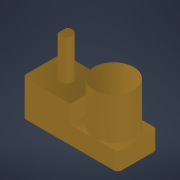
# Autodesk Inventor part: GM1024BY10
Saved by Autodesk Inventor 2022 (Build 260153000, 153)
## iProperties
Created: 2022-04-03
Part Number: GM1024BY10
Material: Bronze, Soft Tin
Document SubType Name: Modeling
Designer: Vinicius Miguel
Density: 8.874 g/cm^3
Appearance: Brass - Satin
Author: Vinicius Miguel
Autodesk Inventor part; units mm, degrees
ref_plane "YZ Plane" through (0, 0, 0) normal (1, 0, 0) x (0, 1, 0)
ref_plane "XZ Plane" through (0, 0, 0) normal (0, 1, 0) x (-1, 0, 0)
ref_plane "XY Plane" through (0, 0, 0) normal (0, 0, 1) x (1, 0, 0)
sketch "Sketch1" plane through (0, 0, 0) normal (0, 1, 0) x (-1, 0, 0)
  circle A0 centre (0, 0) radius 1.5
  dimension "d0" = 3
  constraints: 1 centre point, 1 coincident
  measures "d0" diameter of A0
extrude "Extrusion1" add sketch "Sketch1" along normal blind 10
sketch "Sketch2" plane through (0, 0, 0) normal (0, -1, 0) x (1, 0, 0)
  line L0 (6, 5) -> (-6, 5)
  line L1 (-6, 5) -> (-6, -5)
  line L2 (-6, -5) -> (6, -5)
  line L3 (6, -5) -> (6, 5)
  line L4 (6, 5) -> (-6, -5) construction
  line L5 (-6, 5) -> (6, -5) construction
  point P0 (0, 0)
  point P1 (0, 0)
  point P2 (0, 0)
  point P3 (0, 0)
  dimension "d3" = 10
  dimension "d4" = 12
  constraints: 12 end point, 4 midpoint, 2 coincident, 2 parallel, 1 horizontal, 1 perpendicular
  measures "d3" distance of L0.end L1.end
  measures "d4" distance of L0.start L0.end
extrude "Extrusion2" add sketch "Sketch2" along normal blind 9
sketch "Sketch3" plane through (6, 0, 5) normal (1, 0, 0) x (0, 0, -1)
  line L0 (10, 0) -> (0, 0) projected
  line L1 (0, 0) -> (0, -9) projected
  line L2 (10, -9) -> (0, -9) projected
  line L3 (10, 0) -> (10, -9) projected
  line L4 (0, 0) -> (0, -9) projected
  line L5 (0, -4.5) -> (10, -4.5)
  line L6 (10, 0) -> (10, -9) projected
  point P0 (5, 0)
  point P1 (0, -4.5)
  constraints: 2 end point, 2 midpoint
extrude "Extrusion3" add sketch "Sketch3" along normal blind 12 contours L3 L2 L1 L5
sketch "Sketch4" plane through (6, -4.5, 5) normal (0, 1, 0) x (1, 0, 0)
  line L0 (0, 0) -> (0, 10) projected
  line L1 (0, 0) -> (12, 0) projected
  line L2 (12, 10) -> (12, 0) projected
  line L3 (0, 10) -> (12, 10) projected
  circle A0 centre (6, 5) radius 5
  point P0 (-6, 5)
  point P1 (12, 5)
  point P2 (6, 0)
  dimension "d9" = 10
  constraints: 2 midpoint, 1 centre point, 1 horizontal alignment, 1 vertical alignment
  measures "d9" diameter of A0
extrude "Extrusion4" add sketch "Sketch4" along normal blind 10.5 contours A0
fillet "Fillet1" radius 1 4 edges at (-6, -4.5, 5) (18, -6.75, 5) (18, -6.75, -5) (-6, -4.5, -5)
sketch "Sketch5" plane through (0, 10, 0) normal (0, 1, 0) x (1, 0, 0)
  circle A0 centre (0, 0) radius 1.5 projected
  line L0 (-1, -1.118) -> (-1, 1.118)
  circle A1 centre (0, 0) radius 1.5 projected
  dimension "d13" = 0.5
  constraints: 2 end point, 1 point on circle, 1 vertical, 2 other
extrude "Extrusion5" cut sketch "Sketch5" against normal blind 9 contours L0 A0 picked at (-1.1631, -0.0599)
body "Solid1"
